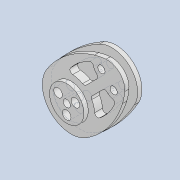
# Autodesk Inventor part: 原動節0
Saved by Autodesk Inventor 2020 (Build 240168000, 168)
## iProperties
Created: 2020-10-27
Part Number: 原動節0
Material: アルミニウム 2014-T4
Document SubType Name: Modeling
Designer: AA19065
Density: 2.8 g/cm^3
Appearance: サテン
Mass: 4.9231 g
Surface Area: 17.3584 cm^2
Volume: 1.75825 cm^3
Author: AA19065
Autodesk Inventor part; units mm, degrees
ref_plane "YZ Plane" through (0, 0, 0) normal (1, 0, 0) x (0, 1, 0)
ref_plane "XZ Plane" through (0, 0, 0) normal (0, 1, 0) x (-1, 0, 0)
ref_plane "XY Plane" through (0, 0, 0) normal (0, 0, 1) x (1, 0, 0)
sketch "スケッチ1" plane through (0, 0, 0) normal (0, 0, 1) x (1, 0, 0)
  line L0 (12.7279, -12.7279) -> (-12.7279, -12.7279) construction
  line L1 (-12.7279, -12.7279) -> (-12.7279, 12.7279) construction
  line L2 (-12.7279, 12.7279) -> (12.7279, 12.7279) construction
  line L3 (12.7279, 12.7279) -> (12.7279, -12.7279) construction
  line L4 (0, 0) -> (-12.7279, -12.7279) construction
  circle A0 centre (0, 0) radius 1.25 construction
  circle A1 centre (-2.1213, 2.1213) radius 1.25
  circle A2 centre (0, 0) radius 6
  circle A3 centre (-12.7279, -12.7279) radius 6
  circle A4 centre (-12.7279, -12.7279) radius 1.25
  circle A5 centre (-12.7279, -16.2279) radius 1.5
  circle A6 centre (-9.6968, -10.9779) radius 1.5
  circle A7 centre (-15.759, -10.9779) radius 1.5
  arc A8 (-0.5224, 5.9772) -> (-18.7051, -12.2055) centre (1.2189, -13.9468) ccw
  arc A9 (-12.2055, -18.7051) -> (5.9772, -0.5224) centre (-13.9468, 1.2189) ccw
  line L5 (-2.1213, 2.1213) -> (0, 0) construction
  circle A10 centre (2.1213, -2.1213) radius 1.25
  dimension "d4" = 18
  dimension "d5" = 2.5
  dimension "d6" = 2.5
  dimension "d8" = 3
  dimension "d9" = 12
  dimension "d10" = 12
  dimension "d11" = 2.5
  dimension "d12" = 3
  dimension "d13" = 360
  dimension "d14" = 3.5
  dimension "d15" = 20
  dimension "d36" = 360
  constraints: 12 end point, 11 centre point, 8 point on circle, 5 coincident, 4 tangent, 1 equal radius, 1 horizontal, 1 perpendicular, 1 point on line, 22 other
  measures "d4" distance of L4.start L0.end
  measures "d5" diameter of A0
  measures "d6" diameter of A1
  measures "d8" distance of A0.centre L5.start
  measures "d9" diameter of A2
  measures "d10" diameter of A3
  measures "d11" diameter of A4
  measures "d12" diameter of A5
  measures "d14" distance of A5.centre A4.centre
  measures "d15" radius of A9
extrude "押し出し1" add sketch "スケッチ1" along normal blind 3
extrude "押し出し2" add sketch "スケッチ1" along normal blind 0.2 contours A5 | A6 | A7
sketch "スケッチ2" plane through (0, 0, 3) normal (0, 0, 1) x (1, 0, 0)
  arc A0 (-12.2055, -18.7051) -> (5.9772, -0.5224) centre (-13.9468, 1.2189) ccw projected
  arc A1 (5.9772, -0.5224) -> (-0.5224, 5.9772) centre (0, 0) ccw projected
  arc A2 (-0.5224, 5.9772) -> (-18.7051, -12.2055) centre (1.2189, -13.9468) ccw projected
  arc A3 (-18.7051, -12.2055) -> (-12.2055, -18.7051) centre (-12.7279, -12.7279) ccw projected
  circle A4 centre (-9.6968, -10.9779) radius 1.5 projected
  circle A5 centre (-12.7279, -12.7279) radius 1.25 projected
  circle A6 centre (-15.759, -10.9779) radius 1.5 projected
  circle A7 centre (-12.7279, -16.2279) radius 1.5 projected
  circle A8 centre (-2.1213, 2.1213) radius 1.25 projected
  circle A9 centre (-12.7279, -12.7279) radius 6
  point P0 (-12.2055, -18.7051)
  point P1 (-18.7051, -12.2055)
  dimension "d21" = 12
  constraints: 1 centre point, 1 coincident
  measures "d21" diameter of A9
extrude "押し出し3" add sketch "スケッチ2" along normal blind 1.5 contours A3 A9
sketch "スケッチ3" plane through (0, 0, 0) normal (0, 0, -1) x (-1, 0, 0)
  arc A0 (-5.9772, -0.5224) -> (12.2055, -18.7051) centre (13.9468, 1.2189) ccw projected
  arc A1 (12.2055, -18.7051) -> (18.7051, -12.2055) centre (12.7279, -12.7279) ccw projected
  arc A2 (18.7051, -12.2055) -> (0.5224, 5.9772) centre (-1.2189, -13.9468) ccw projected
  arc A3 (0.5224, 5.9772) -> (-5.9772, -0.5224) centre (0, 0) ccw projected
  circle A4 centre (12.7279, -12.7279) radius 1.25 projected
  circle A5 centre (2.1213, 2.1213) radius 1.25 projected
  circle A6 centre (12.7279, -12.7279) radius 10
  circle A7 centre (0, 0) radius 9
  point P0 (3.1552, -15.6197)
  point P1 (15.6197, -3.1552)
  point P2 (8.2077, 3.6923)
  point P3 (-3.6923, -8.2077)
  dimension "d24" = 20
  dimension "d28" = 18
  constraints: 2 centre point, 1 coincident
  measures "d24" diameter of A6
  measures "d28" diameter of A7
extrude "押し出し4" add sketch "スケッチ3" against normal up to surface (3 mm away) contours A0 A1 A2 A6
fillet "フィレット1" radius 2 2 edges at (-3.1552, -15.6197, 1.5) (-15.6197, -3.1552, 1.5)
extrude "押し出し5" add sketch "スケッチ3" against normal blind 1.5 contours A0 A7 A2 A3
fillet "フィレット2" radius 2 2 edges at (3.6923, -8.2077, 0.75) (-8.2077, 3.6923, 0.75)
sketch "スケッチ4" plane through (0, 0, 0) normal (0, 0, -1) x (-1, 0, 0)
  circle A0 centre (12.7279, -12.7279) radius 6 projected
  arc A1 (-3.402, -8.7318) -> (2.6127, -15.2594) centre (13.9468, 1.2189) ccw projected
  arc A2 (3.354, -16.2107) -> (2.6127, -15.2594) centre (1.4792, -16.9073) ccw projected
  arc A3 (3.354, -16.2107) -> (16.2107, -3.354) centre (12.7279, -12.7279) ccw projected
  arc A4 (15.2594, -2.6127) -> (16.2107, -3.354) centre (16.9073, -1.4792) ccw projected
  arc A5 (15.2594, -2.6127) -> (8.7318, 3.402) centre (-1.2189, -13.9468) ccw projected
  arc A6 (7.9584, 4.2029) -> (8.7318, 3.402) centre (9.7269, 5.1369) ccw projected
  arc A7 (7.9584, 4.2029) -> (-4.2029, -7.9584) centre (0, 0) ccw projected
  arc A8 (-3.402, -8.7318) -> (-4.2029, -7.9584) centre (-5.1369, -9.7269) ccw projected
  circle A9 centre (12.7279, -12.7279) radius 1.25 projected
  circle A10 centre (2.1213, 2.1213) radius 1.25 projected
  arc A11 (-8.6456, -2.5006) -> (9.0053, -22.0092) centre (20.1732, 5.8346) ccw
  arc A12 (22.0092, -9.0053) -> (2.5006, 8.6456) centre (-5.8346, -20.1732) ccw
  arc A13 (7.9584, 4.2029) -> (-4.2029, -7.9584) centre (0, 0) ccw projected
  arc A14 (3.354, -16.2107) -> (16.2107, -3.354) centre (12.7279, -12.7279) ccw projected
  point P0 (12.2055, -18.7051)
  point P1 (18.7051, -12.2055)
  dimension "d32" = 30
  dimension "d33" = 30
  constraints: 8 point on circle, 4 tangent, 2 centre point
  measures "d32" radius of A11
  measures "d33" radius of A12
sketch "スケッチ5" plane through (0, 0, 3) normal (0, 0, 1) x (1, 0, 0)
  circle A0 centre (-12.7279, -12.7279) radius 6 projected
  arc A1 (-2.6127, -15.2594) -> (5.9772, -0.5224) centre (-13.9468, 1.2189) ccw projected
  arc A2 (5.9772, -0.5224) -> (-0.5224, 5.9772) centre (0, 0) ccw projected
  arc A3 (-0.5224, 5.9772) -> (-15.2594, -2.6127) centre (1.2189, -13.9468) ccw projected
  arc A4 (-16.2107, -3.354) -> (-15.2594, -2.6127) centre (-16.9073, -1.4792) ccw projected
  arc A5 (-16.2107, -3.354) -> (-3.354, -16.2107) centre (-12.7279, -12.7279) ccw projected
  arc A6 (-2.6127, -15.2594) -> (-3.354, -16.2107) centre (-1.4792, -16.9073) ccw projected
  circle A7 centre (-2.1213, 2.1213) radius 1.25 projected
  circle A8 centre (2.1213, -2.1213) radius 1.25 projected
  circle A9 centre (-2.1213, 2.1213) radius 2.75
  circle A10 centre (2.1213, -2.1213) radius 2.75
  arc A11 (-0.3483, 3.9848) -> (-13.6116, -3.7461) centre (1.2189, -13.9468) ccw
  arc A12 (3.9848, -0.3483) -> (-0.3483, 3.9848) centre (0, 0) ccw
  arc A13 (-3.7461, -13.6116) -> (3.9848, -0.3483) centre (-13.9468, 1.2189) ccw
  arc A14 (-3.7461, -13.6116) -> (-5.2288, -15.5142) centre (-1.4792, -16.9073) ccw
  arc A15 (-15.5142, -5.2288) -> (-5.2288, -15.5142) centre (-12.7279, -12.7279) ccw
  arc A16 (-15.5142, -5.2288) -> (-13.6116, -3.7461) centre (-16.9073, -1.4792) ccw
  line L0 (-4.0659, 0.1768) -> (0.1768, -4.0659)
  line L1 (-8.4853, -8.4853) -> (0, 0)
  line L2 (-9.6807, -7.5593) -> (-1.0607, 1.0607)
  line L3 (-7.5593, -9.6807) -> (1.0607, -1.0607)
  circle A17 centre (-12.7279, -12.7279) radius 6 projected
  circle A18 centre (-12.7279, -12.7279) radius 8.2745
  point P0 (-14.4485, -4.6343)
  point P1 (-5.9132, -8.0346)
  point P2 (-4.6343, -14.4485)
  point P3 (3.0486, -4.7103)
  point P4 (-0.8839, -3.0052)
  point P5 (-8.0346, -5.9132)
  point P6 (-3.0052, -0.8839)
  point P7 (-4.7103, 3.0486)
  dimension "d39" = 1.5
  dimension "d40" = 1.5
  dimension "d41" = 2
  dimension "d42" = 1.5
  dimension "d43" = 1.5
  constraints: 15 point on circle, 8 end point, 6 centre point, 2 parallel, 1 perpendicular, 18 other
  measures "d41" radial gap between concentric circles of A3 A11
  measures "d42" distance between parallel lines of L1 L2
  measures "d43" distance between parallel lines of L1 L3
extrude "押し出し6" cut sketch "スケッチ5" against normal blind 2.7 contours L3 L0 A10 A13 A14 A18 | A18 A16 A11 A9 L0 L2
fillet "フィレット3" radius 1.05 8 edges at (-4.7103, 3.0486, 1.65) (3.0486, -4.7103, 1.65) (-4.6343, -14.4485, 1.65) (-14.4485, -4.6343, 1.65) (-8.0346, -5.9132, 1.65) (-5.9132, -8.0346, 1.65) (-3.0052, -0.8839, 1.65) (-0.8839, -3.0052, 1.65)
sketch "スケッチ6" plane through (0, 0, 3) normal (0, 0, 1) x (1, 0, 0)
  arc A0 (-4.474, -12.1451) -> (-5.4999, -8.7001) centre (-12.7279, -12.7279) ccw projected
  arc A1 (-5.3252, -7.4465) -> (-5.4999, -8.7001) centre (-4.5827, -8.189) ccw projected
  line L0 (-5.3252, -7.4465) -> (-1.6263, -3.7477) projected
  arc A2 (-0.1414, -3.7477) -> (-1.6263, -3.7477) centre (-0.8839, -4.4901) ccw projected
  line L1 (-0.1414, -3.7477) -> (0.1768, -4.0659) projected
  arc A3 (0.1768, -4.0659) -> (1.6378, -4.8285) centre (2.1213, -2.1213) ccw projected
  arc A4 (2.4072, -6.3008) -> (1.6378, -4.8285) centre (1.4532, -5.8621) ccw projected
  arc A5 (-2.7749, -12.8945) -> (2.4072, -6.3008) centre (-13.9468, 1.2189) ccw projected
  arc A6 (-4.474, -12.1451) -> (-2.7749, -12.8945) centre (-3.4266, -12.0712) ccw projected
  arc A7 (-12.8945, -2.7749) -> (-12.1451, -4.474) centre (-12.0712, -3.4266) ccw projected
  arc A8 (-6.3008, 2.4072) -> (-12.8945, -2.7749) centre (1.2189, -13.9468) ccw projected
  arc A9 (-4.8285, 1.6378) -> (-6.3008, 2.4072) centre (-5.8621, 1.4532) ccw projected
  arc A10 (-4.8285, 1.6378) -> (-4.0659, 0.1768) centre (-2.1213, 2.1213) ccw projected
  line L2 (-4.0659, 0.1768) -> (-3.7477, -0.1414) projected
  arc A11 (-3.7477, -1.6263) -> (-3.7477, -0.1414) centre (-4.4901, -0.8839) ccw projected
  line L3 (-3.7477, -1.6263) -> (-7.4465, -5.3252) projected
  arc A12 (-8.7001, -5.4999) -> (-7.4465, -5.3252) centre (-8.189, -4.5827) ccw projected
  arc A13 (-8.7001, -5.4999) -> (-12.1451, -4.474) centre (-12.7279, -12.7279) ccw projected
  circle A14 centre (-12.7279, -12.7279) radius 6 projected
  arc A15 (-2.6127, -15.2594) -> (5.9772, -0.5224) centre (-13.9468, 1.2189) ccw projected
  arc A16 (5.9772, -0.5224) -> (-0.5224, 5.9772) centre (0, 0) ccw projected
  arc A17 (-0.5224, 5.9772) -> (-15.2594, -2.6127) centre (1.2189, -13.9468) ccw projected
  arc A18 (-16.2107, -3.354) -> (-15.2594, -2.6127) centre (-16.9073, -1.4792) ccw projected
  arc A19 (-16.2107, -3.354) -> (-3.354, -16.2107) centre (-12.7279, -12.7279) ccw projected
  arc A20 (-2.6127, -15.2594) -> (-3.354, -16.2107) centre (-1.4792, -16.9073) ccw projected
  circle A21 centre (-2.1213, 2.1213) radius 1.25 projected
  circle A22 centre (2.1213, -2.1213) radius 1.25 projected
  arc A23 (-4.5647, 5.1987) -> (-21.1472, -7.3321) centre (4.1107, -23.5196) ccw
  arc A24 (-16.2107, -3.354) -> (-3.354, -16.2107) centre (-12.7279, -12.7279) ccw projected
  arc A25 (-7.3321, -21.1472) -> (5.1987, -4.5647) centre (-23.5196, 4.1107) ccw
  arc A26 (-2.6127, -15.2594) -> (5.9772, -0.5224) centre (-13.9468, 1.2189) ccw projected
  point P0 (-7.3321, -21.1472)
  dimension "d47" = 30
  constraints: 8 point on circle, 4 tangent, 2 centre point, 1 equal radius
  measures "d47" radius of A23
extrude "押し出し7" add sketch "スケッチ6" against normal up to surface (3 mm away) contours A15 A25 A19 A20 | A23 A17 A18 A19
sketch "スケッチ7" plane through (0, 0, 0) normal (0, 0, -1) x (-1, 0, 0)
  circle A0 centre (-2.1213, -2.1213) radius 1.25 projected
  circle A1 centre (2.1213, 2.1213) radius 1.25 projected
  circle A2 centre (12.7279, -12.7279) radius 1.25 projected
  arc A3 (-3.8338, -8.2097) -> (7.3321, -21.1472) centre (23.5196, 4.1107) ccw projected
  arc A4 (7.3321, -21.1472) -> (21.1472, -7.3321) centre (12.7279, -12.7279) ccw projected
  arc A5 (21.1472, -7.3321) -> (8.2097, 3.8338) centre (-4.1107, -23.5196) ccw projected
  arc A6 (7.9584, 4.2029) -> (8.2097, 3.8338) centre (9.7269, 5.1369) ccw projected
  arc A7 (7.9584, 4.2029) -> (-4.2029, -7.9584) centre (0, 0) ccw projected
  arc A8 (-3.8338, -8.2097) -> (-4.2029, -7.9584) centre (-5.1369, -9.7269) ccw projected
  arc A9 (19.4672, -4.9701) -> (4.3528, 7.8774) centre (-19.8293, -35.8859) ccw
  arc A10 (-7.8774, -4.3528) -> (4.9701, -19.4672) centre (35.8859, 19.8293) ccw
  arc A11 (21.1472, -7.3321) -> (8.2097, 3.8338) centre (-4.1107, -23.5196) ccw projected
  arc A12 (7.9584, 4.2029) -> (-4.2029, -7.9584) centre (0, 0) ccw projected
  dimension "d50" = 50
  constraints: 8 point on circle, 4 tangent, 2 centre point, 1 equal radius
  measures "d50" radius of A10
extrude "押し出し8" add sketch "スケッチ7" against normal up to surface (1.5 mm away) contours A3 A10 A7 A8 | A9 A5 A6 A7
equation "\"d4\" = d16"
equation "\"d6\" = d5"
equation "\"d11\" = d6"
equation "\"d33\" = d32"
equation "\"d40\" = d39"
equation "\"d16\" = 18"
